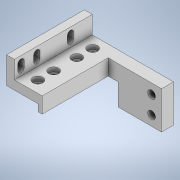
# Autodesk Inventor part: Non_compliant_plate
Saved by Autodesk Inventor 2022.1 (Build 261234000, 234)
## iProperties
Created: 2021-08-01
Part Number: Non_compliant_plate
Material: Generic
Document SubType Name: Modeling
Designer: exllu
Density: 1 g/cm^3
Appearance: Default
Author: exllu
Autodesk Inventor part; units mm, degrees
ref_plane "YZ Plane" through (0, 0, 0) normal (1, 0, 0) x (0, 1, 0)
ref_plane "XZ Plane" through (0, 0, 0) normal (0, 1, 0) x (-1, 0, 0)
ref_plane "XY Plane" through (0, 0, 0) normal (0, 0, 1) x (1, 0, 0)
sketch "Sketch1" plane through (0, 0, 0) normal (0, 1, 0) x (-1, 0, 0)
  line L0 (0, 0) -> (16, 0)
  line L1 (16, 0) -> (16, 40.3)
  line L2 (16, 40.3) -> (0, 40.3)
  line L3 (0, 40.3) -> (0, 0)
  dimension "d0" = 16
  dimension "d1" = 40.3
  constraints: 8 end point, 2 parallel, 1 horizontal, 1 perpendicular
  measures "d0" distance of L2.end L1.end
  measures "d1" distance of L1.end L0.end
extrude "Extrusion1" add sketch "Sketch1" along normal blind 4.5
sketch "Sketch2" plane through (0, 4.5, 0) normal (0, 1, 0) x (1, 0, 0)
  line L0 (0, -40.3) -> (0, 0) projected
  line L1 (0, 0) -> (-6, 0)
  line L2 (0, 0) -> (-16, 0) projected
  line L3 (-6, 0) -> (-6, -5.825)
  line L4 (-6, -5.825) -> (-6, -13.825)
  line L5 (-6, -13.825) -> (-6, -25.475)
  line L6 (-6, -25.475) -> (-6, -33.475)
  circle A0 centre (-6, -33.475) radius 1.05
  circle A1 centre (-6, -25.475) radius 1.05
  circle A2 centre (-6, -13.825) radius 1.05
  circle A3 centre (-6, -5.825) radius 1.05
  dimension "d4" = 6
  dimension "d5" = 5.825
  dimension "d6" = 8
  dimension "d7" = 11.65
  dimension "d8" = 8
  dimension "d9" = 2.1
  dimension "d10" = 2.1
  dimension "d11" = 2.1
  dimension "d12" = 2.1
  constraints: 10 end point, 4 centre point, 4 coincident, 3 point on line, 1 perpendicular, 1 vertical
  measures "d4" distance of L0.end L1.end
  measures "d5" distance of L1.end L3.end
  measures "d6" distance of L3.end L4.end
  measures "d7" distance of L4.end L5.end
  measures "d8" distance of L5.end L6.end
  measures "d9" diameter of A0
  measures "d10" diameter of A1
  measures "d11" diameter of A2
  measures "d12" diameter of A3
extrude "Extrusion2" cut sketch "Sketch2" against normal blind 5
sketch "Sketch3" plane through (0, 4.5, 0) normal (0, 1, 0) x (1, 0, 0)
  circle A0 centre (-6, -5.825) radius 1.05 projected
  circle A1 centre (-6, -5.825) radius 2.5
  circle A2 centre (-6, -13.825) radius 1.05 projected
  circle A3 centre (-6, -13.825) radius 2.5
  circle A4 centre (-6, -25.475) radius 1.05 projected
  circle A5 centre (-6, -25.475) radius 2.5
  circle A6 centre (-6, -33.475) radius 1.05 projected
  circle A7 centre (-6, -33.475) radius 2.5
  point P0 (0, 0)
  dimension "d15" = 5
  dimension "d16" = 5
  dimension "d17" = 5
  dimension "d18" = 5
  constraints: 4 centre point, 4 coincident
  measures "d15" diameter of A1
  measures "d16" diameter of A3
  measures "d17" diameter of A5
  measures "d18" diameter of A7
extrude "Extrusion3" cut sketch "Sketch3" against normal blind 2.2
sketch "Sketch4" plane through (-16, 0, 40.3) normal (0, 0, 1) x (1, 0, 0)
  line L0 (16, 4.5) -> (0, 4.5) projected
  line L1 (0, 0) -> (16, 0)
  line L2 (16, 0) -> (16, 4.5)
  line L3 (16, 4.5) -> (0, 4.5)
  line L4 (0, 4.5) -> (0, 0)
  point P0 (0, 4.5)
  constraints: 8 end point, 2 parallel, 1 horizontal, 1 perpendicular
extrude "Extrusion4" cut sketch "Sketch4" against normal blind 1
sketch "Sketch5" plane through (-16, 0, 39.3) normal (0, 0, 1) x (1, 0, 0)
  line L0 (0, 0) -> (0, 4.5) projected
  line L1 (0, 0) -> (0, 4.5)
  line L2 (0, 4.5) -> (0, 12)
  line L3 (0, 12) -> (4, 12)
  line L4 (4, 12) -> (4, 4.5)
  line L5 (16, 4.5) -> (0, 4.5) projected
  line L6 (4, 4.5) -> (0, 4.5)
  point P0 (16, 0)
  dimension "d23" = 7.5
  dimension "d24" = 4
  constraints: 10 end point, 3 perpendicular, 2 point on line, 1 collinear
  measures "d23" distance of L0.end L2.end
  measures "d24" distance of L2.end L3.end
extrude "Extrusion5" add sketch "Sketch5" against normal blind 39.3
sketch "Sketch6" plane through (-12, 4.5, 39.3) normal (1, 0, 0) x (0, 0, -1)
  line L0 (39.3, 7.5) -> (39.3, 0) projected
  line L1 (39.3, 0) -> (39.3, 3)
  line L2 (39.3, 3) -> (29.9, 3)
  line L3 (28.3, 3) -> (12.9, 3)
  line L4 (11.3, 3) -> (3.3, 3)
  arc A0 (1.7, 3) -> (4.3224, 4.2308) centre (3.3, 3) ccw
  arc A1 (9.7, 3) -> (12.9, 3) centre (11.3, 3) ccw
  arc A2 (26.7, 3) -> (29.9, 3) centre (28.3, 3) ccw
  line L5 (3.3, 3) -> (3.3, 6)
  arc A3 (12.5682, 5.0245) -> (10.0318, 5.0245) centre (11.3, 6) ccw
  line L6 (4.9, 6) -> (4.9, 3)
  line L7 (1.7, 6) -> (1.7, 3)
  arc A4 (4.9, 6) -> (1.7, 6) centre (3.3, 6) ccw
  arc A5 (2.4693, 5) -> (3.3, 4.7) centre (3.3, 6) ccw
  line L8 (11.3, 3) -> (11.3, 3.7)
  line L9 (11.3, 4.3) -> (11.3, 6)
  line L10 (28.3, 3) -> (28.3, 3.7)
  line L11 (9.7, 3) -> (9.7, 6)
  line L12 (12.9, 3) -> (12.9, 6)
  line L13 (28.3, 3) -> (28.3, 6)
  arc A6 (29.9, 6) -> (26.7, 6) centre (28.3, 6) ccw
  line L14 (29.9, 3) -> (29.9, 6)
  line L15 (26.7, 3) -> (26.7, 6)
  point P0 (39.3, -4.5)
  dimension "d27" = 3
  dimension "d28" = 11
  dimension "d29" = 17
  dimension "d30" = 8
  dimension "d36" = 3.2
  dimension "d37" = 3.2
  dimension "d38" = 3.2
  dimension "d39" = 3
  dimension "d40" = 3
  dimension "d43" = 3.2
  dimension "d49" = 3
  dimension "d50" = 3.2
  constraints: 30 end point, 17 point on circle, 7 centre point, 7 point on line, 6 coincident, 6 tangent, 5 vertical, 1 perpendicular
  measures "d27" distance of L0.end L1.end
  measures "d28" distance of L1.end L3.start
  measures "d29" distance of L3.start L4.start
  measures "d30" distance of L4.start L4.end
  measures "d36" diameter of A0
  measures "d37" diameter of A1
  measures "d38" diameter of A2
  measures "d39" distance of L5.start L5.end
  measures "d40" distance of L8.start L9.end
  measures "d43" diameter of A3
  measures "d49" distance of L10.start L13.end
  measures "d50" diameter of A6
extrude "Extrusion6" cut sketch "Sketch6" against normal blind 4.5 contours A0 L7 A4 L6
sketch "Sketch7" plane through (-16, 12, 39.3) normal (0, 1, 0) x (1, 0, 0)
  line L0 (0, 0) -> (0, 39.3) projected
  line L1 (0, 0) -> (4, 0)
  line L2 (4, 0) -> (4, 39.3)
  line L3 (4, 39.3) -> (0, 39.3)
  line L4 (0, 39.3) -> (0, 0)
  point P0 (16, 39.3)
  constraints: 8 end point, 2 parallel, 1 horizontal, 1 perpendicular
extrude "Extrusion7" add sketch "Sketch7" along normal blind 1.5
extrude "Extrusion8" cut sketch "Sketch6" along normal mid plane 3 contours A1 L11 A3 L12 | L15 A6 L14 A2
sketch "Sketch8" plane through (0, 0, 0) normal (1, 0, 0) x (0, 0, -1)
  line L0 (0, 0) -> (0, 4.5) projected
  line L1 (0, 0) -> (0, 4.5)
  line L2 (0, 4.5) -> (0, -3.5)
  line L3 (-39.3, 4.5) -> (0, 4.5) projected
  line L4 (0, 4.5) -> (-39.3, 4.5)
  line L5 (-39.3, 4.5) -> (-39.3, -3.5)
  line L6 (-39.3, 0) -> (-39.3, 13.5) projected
  line L7 (-39.3, -3.5) -> (0, -3.5)
  dimension "d53" = 8
  constraints: 10 end point, 1 collinear, 1 horizontal, 1 perpendicular, 1 point on line, 1 vertical
  measures "d53" distance of L0.end L2.end
extrude "Extrusion9" add sketch "Sketch8" along normal blind 2
sketch "Sketch9" plane through (2, 0, 0) normal (1, 0, 0) x (0, 0, -1)
  line L0 (0, 0) -> (0, 4.5)
  line L1 (0, 4.5) -> (0, -14.5)
  line L2 (0, -14.5) -> (-6, -14.5)
  line L3 (-6, -14.5) -> (-6, 4.5)
  line L4 (-8.325, 4.5) -> (-8.325, 2.3) projected
  line L5 (0, 4.5) -> (-39.3, 4.5) projected
  line L6 (-6, 4.5) -> (0, 4.5)
  dimension "d56" = 19
  dimension "d57" = 6
  constraints: 10 end point, 2 perpendicular, 1 parallel, 1 point on line
  measures "d56" distance of L0.end L1.end
  measures "d57" distance of L1.end L2.end
extrude "Extrusion10" add sketch "Sketch9" along normal blind 27
sketch "Sketch10" plane through (-12, 13.5, 0) normal (0, 0, -1) x (-1, 0, 0)
  line L0 (-14, -9) -> (-41, -9) projected
  line L1 (-41, -9) -> (-36, -9)
  line L2 (-36, -9) -> (-36, -14)
  circle A0 centre (-36, -14) radius 1.9305
  line L3 (-14, -28) -> (-41, -28) projected
  line L4 (-41, -28) -> (-36, -28)
  line L5 (-36, -28) -> (-36, -23)
  circle A1 centre (-36, -23) radius 1.9305
  point P0 (-12, -13.5)
  dimension "d60" = 5
  dimension "d61" = 5
  dimension "d62" = 3.861
  dimension "d63" = 5
  dimension "d64" = 5
  dimension "d65" = 3.861
  constraints: 8 end point, 2 centre point, 2 coincident, 2 perpendicular, 2 point on line
  measures "d60" distance of L0.end L1.end
  measures "d61" distance of L1.end L2.end
  measures "d62" diameter of A0
  measures "d63" distance of L3.end L4.end
  measures "d64" distance of L4.end L5.end
  measures "d65" diameter of A1
extrude "Extrusion11" cut sketch "Sketch10" against normal blind 20
sketch "Sketch11" plane through (-12, 13.5, 0) normal (0, 0, -1) x (-1, 0, 0)
  line L0 (-14, -28) -> (-41, -28) projected
  line L1 (-14, -28) -> (-19, -28)
  line L2 (-19, -28) -> (-19, -17)
  line L3 (-19, -17) -> (-14, -17)
  line L4 (-14, -17) -> (-14, -28)
  point P0 (-12, -13.5)
  point P1 (-19, -28)
  dimension "d68" = 5
  dimension "d69" = 11
  constraints: 8 end point, 2 parallel, 1 horizontal, 1 perpendicular
  measures "d68" distance of L2.end L3.end
  measures "d69" distance of L1.end L2.end
extrude "Extrusion12" cut sketch "Sketch11" against normal blind 25
sketch "Sketch12" plane through (-13.5, 4.5, 39.3) normal (1, 0, 0) x (0, 0, -1)
  arc A0 (12.9, 6) -> (9.7, 6) centre (11.3, 6) ccw projected
  circle A1 centre (11.3, 6) radius 1.6
  arc A2 (9.7, 3) -> (12.9, 3) centre (11.3, 3) ccw projected
  circle A3 centre (11.3, 3) radius 1.6
  line L0 (9.7, 3) -> (9.7, 6) projected
  line L1 (9.7, 6) -> (9.7, 3)
  line L2 (12.9, 6) -> (12.9, 3) projected
  line L3 (12.9, 6) -> (12.9, 3)
  arc A4 (26.7, 3) -> (29.9, 3) centre (28.3, 3) ccw projected
  line L4 (11.3, 3) -> (28.3, 3)
  line L5 (28.3, 3) -> (19.8, 3)
  line L6 (19.8, 3) -> (19.8, 4.3)
  arc A5 (29.9, 6) -> (26.7, 6) centre (28.3, 6) ccw
  circle A6 centre (28.3, 6) radius 1.6
  circle A7 centre (28.3, 3) radius 1.6
  line L7 (29.9, 3) -> (29.9, 6)
  line L8 (29.9, 6) -> (29.9, 3)
  line L9 (26.7, 6) -> (26.7, 3)
  line L10 (26.7, 6) -> (26.7, 3)
  point P0 (39.3, -4.5)
  constraints: 18 end point, 5 symmetric about line, 3 centre point, 3 coincident, 3 vertical, 2 horizontal alignment, 2 point on circle, 1 collinear, 1 horizontal, 1 midpoint, 1 tangent, 6 other
extrude "Extrusion13" cut sketch "Sketch12" against normal blind 3
sketch "Sketch13" plane through (-12, 4.5, 39.3) normal (1, 0, 0) x (0, 0, -1)
  arc A0 (4.9, 6) -> (3.8568, 7.5) centre (3.3, 6) ccw projected
  circle A1 centre (3.3, 6) radius 1.6
  point P0 (39.3, -4.5)
  point P1 (4.9, 6)
  dimension "d74" = 3.2
  constraints: 1 centre point, 1 coincident
  measures "d74" diameter of A1
extrude "Extrusion14" cut sketch "Sketch13" along normal mid plane 8
body "Solid1"
